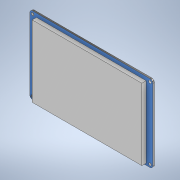
# Autodesk Inventor part: Tela Led
Saved by Autodesk Inventor 2020 (Build 240168000, 168)
## iProperties
Created: 2019-09-20
Part Number: Tela Led
Material: Generic
Document SubType Name: Modeling
Designer: Acer
Density: 1 g/cm^3
Appearance: Default
Author: Acer
Autodesk Inventor part; units mm, degrees
ref_plane "YZ Plane" through (0, 0, 0) normal (1, 0, 0) x (0, 1, 0)
ref_plane "XZ Plane" through (0, 0, 0) normal (0, 1, 0) x (-1, 0, 0)
ref_plane "XY Plane" through (0, 0, 0) normal (0, 0, 1) x (1, 0, 0)
sketch "Sketch1" plane through (0, 0, 0) normal (0, 0, 1) x (1, 0, 0)
  line L0 (-66.75, 41.75) -> (66.75, 41.75)
  line L1 (66.75, 41.75) -> (66.75, -41.75)
  line L2 (66.75, -41.75) -> (-66.75, -41.75)
  line L3 (-66.75, -41.75) -> (-66.75, 41.75)
  line L4 (-66.75, 41.75) -> (66.75, -41.75) construction
  line L5 (66.75, 41.75) -> (-66.75, -41.75) construction
  circle A0 centre (-63.75, 38.75) radius 1.5
  circle A1 centre (63.75, 38.75) radius 1.5
  circle A2 centre (63.75, -38.75) radius 1.5
  circle A3 centre (-63.75, -38.75) radius 1.5
  point P0 (0, 0)
  dimension "d0" = 133.5
  dimension "d1" = 83.5
  dimension "d2" = 3
  dimension "d3" = 3
  dimension "d4" = 3
  dimension "d5" = 3
  dimension "d6" = 3
  dimension "d7" = 3
  dimension "d8" = 3
  dimension "d9" = 3
  dimension "d10" = 3
  dimension "d11" = 3
  dimension "d12" = 3
  dimension "d13" = 3
  constraints: 12 end point, 4 centre point, 2 midpoint, 2 parallel, 1 horizontal, 1 perpendicular
  measures "d0" distance of L1.end L2.end
  measures "d1" distance of L0.end L1.end
  measures "d2" diameter of A0
  measures "d3" diameter of A1
  measures "d4" diameter of A2
  measures "d5" diameter of A3
  measures "d6" distance from line of L3 A0.centre
  measures "d7" distance from line of L0 A0.centre
  measures "d8" distance from line of L1 A1.centre
  measures "d9" distance from line of L0 A1.centre
  measures "d10" distance from line of L2 A2.centre
  measures "d11" distance from line of L1 A2.centre
  measures "d12" distance from line of L2 A3.centre
  measures "d13" distance from line of L3 A3.centre
extrude "Extrusion1" add sketch "Sketch1" along normal blind 1.75
fillet "Fillet1" radius 3 4 edges at (66.75, 41.75, 0.875) (-66.75, 41.75, 0.875) (66.75, -41.75, 0.875) (-66.75, -41.75, 0.875)
sketch "Sketch2" plane through (0, 0, 1.75) normal (0, 0, 1) x (1, 0, 0)
  line L0 (-59.5, 37.75) -> (59.5, 37.75)
  line L1 (59.5, 37.75) -> (59.5, -39.75)
  line L2 (59.5, -39.75) -> (-59.5, -39.75)
  line L3 (-59.5, -39.75) -> (-59.5, 37.75)
  line L4 (-59.5, 37.75) -> (59.5, -39.75) construction
  line L5 (59.5, 37.75) -> (-59.5, -39.75) construction
  line L6 (63.75, 41.75) -> (-63.75, 41.75) projected
  point P0 (0, 0)
  point P1 (0, -1)
  dimension "d17" = 0
  dimension "d19" = 77.5
  dimension "d20" = 4
  dimension "d21" = 119
  constraints: 12 end point, 2 midpoint, 2 parallel, 1 horizontal, 1 perpendicular
  measures "d17" horizontal distance of point (0, 0) point (0, -1)
  measures "d19" distance of L0.end L1.end
  measures "d20" distance between parallel lines of L6 L0
  measures "d21" distance of L1.end L2.end
extrude "Extrusion2" add sketch "Sketch2" along normal blind 4.65
equation "\"d8\" = d6"
equation "\"d9\" = d7"
equation "\"d10\" = d7"
equation "\"d11\" = d6"
equation "\"d12\" = d6"
equation "\"d13\" = d6"
body "Solid1"
